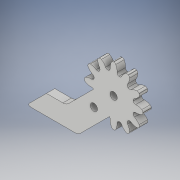
# Autodesk Inventor part: 齒輪
Saved by Autodesk Inventor 2019 (Build 230136000, 136)
## iProperties
Created: 2022-01-10
Part Number: 齒輪
Material: 一般
Document SubType Name: Modeling
Designer: 10617
Density: 1 g/cm^3
Appearance: 預設
Author: 10617
Autodesk Inventor part; units mm, degrees
ref_plane "YZ Plane" through (0, 0, 0) normal (1, 0, 0) x (0, 1, 0)
ref_plane "XZ Plane" through (0, 0, 0) normal (0, 1, 0) x (-1, 0, 0)
ref_plane "XY Plane" through (0, 0, 0) normal (0, 0, 1) x (1, 0, 0)
sketch "草圖1" plane through (0, 0, 0) normal (0, 0, 1) x (1, 0, 0)
  line L0 (35.5372, 27.5707) -> (35.6541, 27.5031)
  spline S0 degree 3 poles (35.5372, 27.5707) (35.2822, 27.7157) (34.9682, 27.7095) (34.7191, 27.5545) knots 0 0 0 0 1 1 1 1
  line L1 (35.5372, 27.5707) -> (35.2822, 27.7157) construction
  line L2 (35.2822, 27.7157) -> (34.9682, 27.7095) construction
  line L3 (34.9682, 27.7095) -> (34.7191, 27.5545) construction
  spline S1 degree 3 poles (32.2222, 25.4467) (32.622, 25.3397) (33.0418, 25.5302) (33.2243, 25.9019) knots 0.333333 0.333333 0.333333 0.333333 1 1 1 1
  line L4 (32.2222, 25.4467) -> (32.622, 25.3397) construction
  line L5 (32.622, 25.3397) -> (33.0418, 25.5302) construction
  line L6 (33.0418, 25.5302) -> (33.2243, 25.9019) construction
  spline S2 degree 3 poles (34.7191, 27.5545) (34.0759, 27.1545) (33.558, 26.5819) (33.2243, 25.9019) knots 0 0 0 0 1 1 1 1
  line L7 (34.7191, 27.5545) -> (34.0759, 27.1545) construction
  line L8 (34.0759, 27.1545) -> (33.558, 26.5819) construction
  line L9 (33.558, 26.5819) -> (33.2243, 25.9019) construction
  spline S3 degree 3 poles (31.582, 26.3419) (31.5542, 25.929) (31.8224, 25.5539) (32.2222, 25.4467) knots 0 0 0 0 0.333333 0.333333 0.333333 0.333333
  line L10 (31.582, 26.3419) -> (31.5542, 25.929) construction
  line L11 (31.5542, 25.929) -> (31.8224, 25.5539) construction
  line L12 (31.8224, 25.5539) -> (32.2222, 25.4467) construction
  spline S4 degree 3 poles (31.582, 26.3419) (31.6329, 27.0977) (31.4707, 27.8525) (31.1137, 28.5206) knots 0 0 0 0 1 1 1 1
  line L13 (31.582, 26.3419) -> (31.6329, 27.0977) construction
  line L14 (31.6329, 27.0977) -> (31.4707, 27.8525) construction
  line L15 (31.4707, 27.8525) -> (31.1137, 28.5206) construction
  spline S5 degree 3 poles (28.4693, 25.4467) (28.8691, 25.5539) (29.1373, 25.9289) (29.1096, 26.3419) knots 0.333333 0.333333 0.333333 0.333333 1 1 1 1
  line L16 (28.4693, 25.4467) -> (28.8691, 25.5539) construction
  line L17 (28.8691, 25.5539) -> (29.1373, 25.9289) construction
  line L18 (29.1373, 25.9289) -> (29.1096, 26.3419) construction
  spline S6 degree 3 poles (31.1137, 28.5206) (30.9755, 28.7793) (30.7066, 28.9417) (30.4132, 28.9436) knots 0 0 0 0 1 1 1 1
  line L19 (31.1137, 28.5206) -> (30.9755, 28.7793) construction
  line L20 (30.9755, 28.7793) -> (30.7066, 28.9417) construction
  line L21 (30.7066, 28.9417) -> (30.4132, 28.9436) construction
  spline S7 degree 3 poles (30.4132, 28.9436) (30.3683, 28.9439) (30.3233, 28.9439) (30.2782, 28.9436) knots 0 0 0 0 1 1 1 1
  line L22 (30.4132, 28.9436) -> (30.3683, 28.9439) construction
  line L23 (30.3683, 28.9439) -> (30.3233, 28.9439) construction
  line L24 (30.3233, 28.9439) -> (30.2782, 28.9436) construction
  spline S8 degree 3 poles (30.2782, 28.9436) (29.9849, 28.9418) (29.716, 28.7794) (29.5778, 28.5207) knots 0 0 0 0 1 1 1 1
  line L25 (30.2782, 28.9436) -> (29.9849, 28.9418) construction
  line L26 (29.9849, 28.9418) -> (29.716, 28.7794) construction
  line L27 (29.716, 28.7794) -> (29.5778, 28.5207) construction
  spline S9 degree 3 poles (29.5778, 28.5207) (29.2209, 27.8526) (29.0586, 27.0977) (29.1096, 26.3419) knots 0 0 0 0 1 1 1 1
  line L28 (29.5778, 28.5207) -> (29.2209, 27.8526) construction
  line L29 (29.2209, 27.8526) -> (29.0586, 27.0977) construction
  line L30 (29.0586, 27.0977) -> (29.1096, 26.3419) construction
  spline S10 degree 3 poles (27.4673, 25.9019) (27.6497, 25.5303) (28.0695, 25.3396) (28.4693, 25.4467) knots 0 0 0 0 0.333333 0.333333 0.333333 0.333333
  line L31 (27.4673, 25.9019) -> (27.6497, 25.5303) construction
  line L32 (27.6497, 25.5303) -> (28.0695, 25.3396) construction
  line L33 (28.0695, 25.3396) -> (28.4693, 25.4467) construction
  spline S11 degree 3 poles (27.4673, 25.9019) (27.1335, 26.5819) (26.6157, 27.1545) (25.9725, 27.5545) knots 0 0 0 0 1 1 1 1
  line L34 (27.4673, 25.9019) -> (27.1335, 26.5819) construction
  line L35 (27.1335, 26.5819) -> (26.6157, 27.1545) construction
  line L36 (26.6157, 27.1545) -> (25.9725, 27.5545) construction
  spline S12 degree 3 poles (24.6423, 26.7866) (24.6672, 26.0295) (24.9041, 25.2947) (25.3261, 24.6657) knots 0 0 0 0 1 1 1 1
  line L37 (24.6423, 26.7866) -> (24.6672, 26.0295) construction
  line L38 (24.6672, 26.0295) -> (24.9041, 25.2947) construction
  line L39 (24.9041, 25.2947) -> (25.3261, 24.6657) construction
  spline S13 degree 3 poles (25.9725, 27.5545) (25.7233, 27.7095) (25.4095, 27.7156) (25.1544, 27.5707) knots 0 0 0 0 1 1 1 1
  line L40 (25.9725, 27.5545) -> (25.7233, 27.7095) construction
  line L41 (25.7233, 27.7095) -> (25.4095, 27.7156) construction
  line L42 (25.4095, 27.7156) -> (25.1544, 27.5707) construction
  spline S14 degree 3 poles (25.1544, 27.5707) (25.1152, 27.5484) (25.0762, 27.5259) (25.0374, 27.5031) knots 0 0 0 0 1 1 1 1
  line L43 (25.1544, 27.5707) -> (25.1152, 27.5484) construction
  line L44 (25.1152, 27.5484) -> (25.0762, 27.5259) construction
  line L45 (25.0762, 27.5259) -> (25.0374, 27.5031) construction
  spline S15 degree 3 poles (25.0374, 27.5031) (24.7843, 27.3548) (24.6326, 27.0798) (24.6423, 26.7866) knots 0 0 0 0 1 1 1 1
  line L46 (25.0374, 27.5031) -> (24.7843, 27.3548) construction
  line L47 (24.7843, 27.3548) -> (24.6326, 27.0798) construction
  line L48 (24.6326, 27.0798) -> (24.6423, 26.7866) construction
  spline S16 degree 3 poles (36.0492, 26.7866) (36.0589, 27.0798) (35.9071, 27.3547) (35.6541, 27.5031) knots 0 0 0 0 1 1 1 1
  line L49 (36.0492, 26.7866) -> (36.0589, 27.0798) construction
  line L50 (36.0589, 27.0798) -> (35.9071, 27.3547) construction
  line L51 (35.9071, 27.3547) -> (35.6541, 27.5031) construction
  spline S17 degree 3 poles (32.2222, 11.4409) (31.8224, 11.3337) (31.5542, 10.9586) (31.582, 10.5457) knots 0.333333 0.333333 0.333333 0.333333 1 1 1 1
  line L52 (32.2222, 11.4409) -> (31.8224, 11.3337) construction
  line L53 (31.8224, 11.3337) -> (31.5542, 10.9586) construction
  line L54 (31.5542, 10.9586) -> (31.582, 10.5457) construction
  spline S18 degree 3 poles (33.2242, 10.9857) (33.0418, 11.3573) (32.622, 11.548) (32.2222, 11.4409) knots 0 0 0 0 0.333333 0.333333 0.333333 0.333333
  line L55 (33.2242, 10.9857) -> (33.0418, 11.3573) construction
  line L56 (33.0418, 11.3573) -> (32.622, 11.548) construction
  line L57 (32.622, 11.548) -> (32.2222, 11.4409) construction
  spline S19 degree 3 poles (33.2242, 10.9857) (33.558, 10.3057) (34.0759, 9.7332) (34.7191, 9.3331) knots 0 0 0 0 1 1 1 1
  line L58 (33.2242, 10.9857) -> (33.558, 10.3057) construction
  line L59 (33.558, 10.3057) -> (34.0759, 9.7332) construction
  line L60 (34.0759, 9.7332) -> (34.7191, 9.3331) construction
  spline S20 degree 3 poles (34.7191, 9.3331) (34.9682, 9.178) (35.2822, 9.172) (35.5372, 9.317) knots 0 0 0 0 1 1 1 1
  line L61 (34.7191, 9.3331) -> (34.9682, 9.178) construction
  line L62 (34.9682, 9.178) -> (35.2822, 9.172) construction
  line L63 (35.2822, 9.172) -> (35.5372, 9.317) construction
  spline S21 degree 3 poles (35.5372, 9.317) (35.5763, 9.3393) (35.6153, 9.3617) (35.6541, 9.3845) knots 0 0 0 0 1 1 1 1
  line L64 (35.5372, 9.317) -> (35.5763, 9.3393) construction
  line L65 (35.5763, 9.3393) -> (35.6153, 9.3617) construction
  line L66 (35.6153, 9.3617) -> (35.6541, 9.3845) construction
  spline S22 degree 3 poles (35.6541, 9.3845) (35.9073, 9.5329) (36.0589, 9.8078) (36.0492, 10.101) knots 0 0 0 0 1 1 1 1
  line L67 (35.6541, 9.3845) -> (35.9073, 9.5329) construction
  line L68 (35.9073, 9.5329) -> (36.0589, 9.8078) construction
  line L69 (36.0589, 9.8078) -> (36.0492, 10.101) construction
  spline S23 degree 3 poles (36.0492, 10.101) (36.0243, 10.8581) (35.7874, 11.5929) (35.3654, 12.2219) knots 0 0 0 0 1 1 1 1
  line L70 (36.0492, 10.101) -> (36.0243, 10.8581) construction
  line L71 (36.0243, 10.8581) -> (35.7874, 11.5929) construction
  line L72 (35.7874, 11.5929) -> (35.3654, 12.2219) construction
  spline S24 degree 3 poles (35.4723, 13.3172) (35.1796, 13.0246) (35.1348, 12.5657) (35.3654, 12.2219) knots 0.333333 0.333333 0.333333 0.333333 1 1 1 1
  line L73 (35.4723, 13.3172) -> (35.1796, 13.0246) construction
  line L74 (35.1796, 13.0246) -> (35.1348, 12.5657) construction
  line L75 (35.1348, 12.5657) -> (35.3654, 12.2219) construction
  spline S25 degree 3 poles (36.5676, 13.4242) (36.2239, 13.6547) (35.7651, 13.61) (35.4723, 13.3172) knots 0 0 0 0 0.333333 0.333333 0.333333 0.333333
  line L76 (36.5676, 13.4242) -> (36.2239, 13.6547) construction
  line L77 (36.2239, 13.6547) -> (35.7651, 13.61) construction
  line L78 (35.7651, 13.61) -> (35.4723, 13.3172) construction
  spline S26 degree 3 poles (36.5676, 13.4242) (37.1967, 13.0022) (37.9315, 12.7653) (38.6886, 12.7403) knots 0 0 0 0 1 1 1 1
  line L79 (36.5676, 13.4242) -> (37.1967, 13.0022) construction
  line L80 (37.1967, 13.0022) -> (37.9315, 12.7653) construction
  line L81 (37.9315, 12.7653) -> (38.6886, 12.7403) construction
  spline S27 degree 3 poles (38.6886, 12.7403) (38.9818, 12.7307) (39.2567, 12.8824) (39.405, 13.1354) knots 0 0 0 0 1 1 1 1
  line L82 (38.6886, 12.7403) -> (38.9818, 12.7307) construction
  line L83 (38.9818, 12.7307) -> (39.2567, 12.8824) construction
  line L84 (39.2567, 12.8824) -> (39.405, 13.1354) construction
  spline S28 degree 3 poles (39.405, 13.1354) (39.4279, 13.1743) (39.4504, 13.2133) (39.4726, 13.2524) knots 0 0 0 0 1 1 1 1
  line L85 (39.405, 13.1354) -> (39.4279, 13.1743) construction
  line L86 (39.4279, 13.1743) -> (39.4504, 13.2133) construction
  line L87 (39.4504, 13.2133) -> (39.4726, 13.2524) construction
  spline S29 degree 3 poles (39.4726, 13.2524) (39.6177, 13.5074) (39.6115, 13.8213) (39.4565, 14.0705) knots 0 0 0 0 1 1 1 1
  line L88 (39.4726, 13.2524) -> (39.6177, 13.5074) construction
  line L89 (39.6177, 13.5074) -> (39.6115, 13.8213) construction
  line L90 (39.6115, 13.8213) -> (39.4565, 14.0705) construction
  spline S30 degree 3 poles (39.4565, 14.0705) (39.0564, 14.7137) (38.4838, 15.2316) (37.8039, 15.5653) knots 0 0 0 0 1 1 1 1
  line L91 (39.4565, 14.0705) -> (39.0564, 14.7137) construction
  line L92 (39.0564, 14.7137) -> (38.4838, 15.2316) construction
  line L93 (38.4838, 15.2316) -> (37.8039, 15.5653) construction
  spline S31 degree 3 poles (37.3487, 16.5674) (37.2416, 16.1675) (37.4323, 15.7477) (37.8039, 15.5653) knots 0.333333 0.333333 0.333333 0.333333 1 1 1 1
  line L94 (37.3487, 16.5674) -> (37.2416, 16.1675) construction
  line L95 (37.2416, 16.1675) -> (37.4323, 15.7477) construction
  line L96 (37.4323, 15.7477) -> (37.8039, 15.5653) construction
  spline S32 degree 3 poles (35.3655, 24.6657) (35.1348, 24.3219) (35.1796, 23.863) (35.4722, 23.5704) knots 0 0 0 0 0.333333 0.333333 0.333333 0.333333
  line L97 (35.3655, 24.6657) -> (35.1348, 24.3219) construction
  line L98 (35.1348, 24.3219) -> (35.1796, 23.863) construction
  line L99 (35.1796, 23.863) -> (35.4722, 23.5704) construction
  spline S33 degree 3 poles (35.4722, 23.5704) (35.765, 23.2776) (36.2238, 23.2329) (36.5676, 23.4635) knots 0.333333 0.333333 0.333333 0.333333 1 1 1 1
  line L100 (35.4722, 23.5704) -> (35.765, 23.2776) construction
  line L101 (35.765, 23.2776) -> (36.2238, 23.2329) construction
  line L102 (36.2238, 23.2329) -> (36.5676, 23.4635) construction
  spline S34 degree 3 poles (38.6885, 24.1473) (37.9315, 24.1224) (37.1967, 23.8855) (36.5676, 23.4635) knots 0 0 0 0 1 1 1 1
  line L103 (38.6885, 24.1473) -> (37.9315, 24.1224) construction
  line L104 (37.9315, 24.1224) -> (37.1967, 23.8855) construction
  line L105 (37.1967, 23.8855) -> (36.5676, 23.4635) construction
  spline S35 degree 3 poles (39.4051, 23.7522) (39.2566, 24.0052) (38.9818, 24.157) (38.6885, 24.1473) knots 0 0 0 0 1 1 1 1
  line L106 (39.4051, 23.7522) -> (39.2566, 24.0052) construction
  line L107 (39.2566, 24.0052) -> (38.9818, 24.157) construction
  line L108 (38.9818, 24.157) -> (38.6885, 24.1473) construction
  spline S36 degree 3 poles (37.8039, 21.3223) (37.4322, 21.1399) (37.2416, 20.7201) (37.3487, 20.3203) knots 0 0 0 0 0.333333 0.333333 0.333333 0.333333
  line L109 (37.8039, 21.3223) -> (37.4322, 21.1399) construction
  line L110 (37.4322, 21.1399) -> (37.2416, 20.7201) construction
  line L111 (37.2416, 20.7201) -> (37.3487, 20.3203) construction
  spline S37 degree 3 poles (39.4726, 23.6353) (39.4504, 23.6744) (39.4278, 23.7133) (39.4051, 23.7522) knots 0 0 0 0 1 1 1 1
  line L112 (39.4726, 23.6353) -> (39.4504, 23.6744) construction
  line L113 (39.4504, 23.6744) -> (39.4278, 23.7133) construction
  line L114 (39.4278, 23.7133) -> (39.4051, 23.7522) construction
  spline S38 degree 3 poles (39.4565, 22.8171) (39.6114, 23.0663) (39.6177, 23.3802) (39.4726, 23.6353) knots 0 0 0 0 1 1 1 1
  line L115 (39.4565, 22.8171) -> (39.6114, 23.0663) construction
  line L116 (39.6114, 23.0663) -> (39.6177, 23.3802) construction
  line L117 (39.6177, 23.3802) -> (39.4726, 23.6353) construction
  spline S39 degree 3 poles (37.3487, 20.3203) (37.4558, 19.9204) (37.8309, 19.6522) (38.2439, 19.6801) knots 0.333333 0.333333 0.333333 0.333333 1 1 1 1
  line L118 (37.3487, 20.3203) -> (37.4558, 19.9204) construction
  line L119 (37.4558, 19.9204) -> (37.8309, 19.6522) construction
  line L120 (37.8309, 19.6522) -> (38.2439, 19.6801) construction
  spline S40 degree 3 poles (37.8039, 21.3223) (38.4838, 21.6561) (39.0564, 22.174) (39.4565, 22.8171) knots 0 0 0 0 1 1 1 1
  line L121 (37.8039, 21.3223) -> (38.4838, 21.6561) construction
  line L122 (38.4838, 21.6561) -> (39.0564, 22.174) construction
  line L123 (39.0564, 22.174) -> (39.4565, 22.8171) construction
  spline S41 degree 3 poles (40.4226, 19.2117) (39.7545, 19.5687) (38.9996, 19.731) (38.2439, 19.6801) knots 0 0 0 0 1 1 1 1
  line L124 (40.4226, 19.2117) -> (39.7545, 19.5687) construction
  line L125 (39.7545, 19.5687) -> (38.9996, 19.731) construction
  line L126 (38.9996, 19.731) -> (38.2439, 19.6801) construction
  spline S42 degree 3 poles (40.8455, 18.3762) (40.8458, 18.4213) (40.8458, 18.4663) (40.8455, 18.5113) knots 0 0 0 0 1 1 1 1
  line L127 (40.8455, 18.3762) -> (40.8458, 18.4213) construction
  line L128 (40.8458, 18.4213) -> (40.8458, 18.4663) construction
  line L129 (40.8458, 18.4663) -> (40.8455, 18.5113) construction
  spline S43 degree 3 poles (40.8455, 18.5113) (40.8436, 18.8047) (40.6813, 19.0735) (40.4226, 19.2117) knots 0 0 0 0 1 1 1 1
  line L130 (40.8455, 18.5113) -> (40.8436, 18.8047) construction
  line L131 (40.8436, 18.8047) -> (40.6813, 19.0735) construction
  line L132 (40.6813, 19.0735) -> (40.4226, 19.2117) construction
  spline S44 degree 3 poles (40.4226, 17.6758) (40.6814, 17.8141) (40.8437, 18.0829) (40.8455, 18.3762) knots 0 0 0 0 1 1 1 1
  line L133 (40.4226, 17.6758) -> (40.6814, 17.8141) construction
  line L134 (40.6814, 17.8141) -> (40.8437, 18.0829) construction
  line L135 (40.8437, 18.0829) -> (40.8455, 18.3762) construction
  spline S45 degree 3 poles (38.2439, 17.2076) (38.9996, 17.1567) (39.7545, 17.3189) (40.4226, 17.6758) knots 0 0 0 0 1 1 1 1
  line L136 (38.2439, 17.2076) -> (38.9996, 17.1567) construction
  line L137 (38.9996, 17.1567) -> (39.7545, 17.3189) construction
  line L138 (39.7545, 17.3189) -> (40.4226, 17.6758) construction
  spline S46 degree 3 poles (38.2439, 17.2076) (37.8309, 17.2353) (37.4559, 16.9672) (37.3487, 16.5674) knots 0 0 0 0 0.333333 0.333333 0.333333 0.333333
  line L139 (38.2439, 17.2076) -> (37.8309, 17.2353) construction
  line L140 (37.8309, 17.2353) -> (37.4559, 16.9672) construction
  line L141 (37.4559, 16.9672) -> (37.3487, 16.5674) construction
  spline S47 degree 3 poles (35.3655, 24.6657) (35.7875, 25.2947) (36.0243, 26.0295) (36.0492, 26.7866) knots 0 0 0 0 1 1 1 1
  line L142 (35.3655, 24.6657) -> (35.7875, 25.2947) construction
  line L143 (35.7875, 25.2947) -> (36.0243, 26.0295) construction
  line L144 (36.0243, 26.0295) -> (36.0492, 26.7866) construction
  arc A0 (12.1679, 7.1654) -> (14.2893, 8.0441) centre (12.1679, 10.1655) ccw
  arc A1 (0.0524, 0.9447) -> (0.4048, 0.0944) centre (0.4031, 0.5919) ccw
  arc A2 (16.4106, 0.0943) -> (18.5319, 0.9731) centre (16.4105, 3.0945) ccw
  line L145 (14.2893, 8.0441) -> (23.1584, 16.9132)
  line L146 (6.2687, 7.1655) -> (12.1679, 7.1654)
  line L147 (6.2687, 7.1655) -> (0.0524, 0.9447)
  line L148 (0.4048, 0.0944) -> (16.4106, 0.0943)
  line L149 (18.5319, 0.9731) -> (28.8152, 11.2564)
  spline S48 degree 3 poles (30.2783, 7.944) (30.3232, 7.9437) (30.3683, 7.9438) (30.4133, 7.944) knots 0 0 0 0 1 1 1 1
  line L150 (30.2783, 7.944) -> (30.3232, 7.9437) construction
  line L151 (30.3232, 7.9437) -> (30.3683, 7.9438) construction
  line L152 (30.3683, 7.9438) -> (30.4133, 7.944) construction
  spline S49 degree 3 poles (30.4133, 7.944) (30.7067, 7.9459) (30.9755, 8.1082) (31.1138, 8.367) knots 0 0 0 0 1 1 1 1
  line L153 (30.4133, 7.944) -> (30.7067, 7.9459) construction
  line L154 (30.7067, 7.9459) -> (30.9755, 8.1082) construction
  line L155 (30.9755, 8.1082) -> (31.1138, 8.367) construction
  spline S50 degree 3 poles (31.1138, 8.367) (31.4707, 9.0351) (31.6329, 9.79) (31.582, 10.5457) knots 0 0 0 0 1 1 1 1
  line L156 (31.1138, 8.367) -> (31.4707, 9.0351) construction
  line L157 (31.4707, 9.0351) -> (31.6329, 9.79) construction
  line L158 (31.6329, 9.79) -> (31.582, 10.5457) construction
  circle A3 centre (23.2746, 11.3728) radius 1.3
  spline S51 degree 3 poles (29.1096, 10.5457) (29.1277, 10.8155) (29.0188, 11.0784) (28.8152, 11.2564) knots 0 0 0 0 1 1 1 1
  line L159 (29.1096, 10.5457) -> (29.1277, 10.8155) construction
  line L160 (29.1277, 10.8155) -> (29.0188, 11.0784) construction
  line L161 (29.0188, 11.0784) -> (28.8152, 11.2564) construction
  spline S52 degree 3 poles (29.5778, 8.367) (29.716, 8.1083) (29.9849, 7.9459) (30.2783, 7.944) knots 0 0 0 0 1 1 1 1
  line L162 (29.5778, 8.367) -> (29.716, 8.1083) construction
  line L163 (29.716, 8.1083) -> (29.9849, 7.9459) construction
  line L164 (29.9849, 7.9459) -> (30.2783, 7.944) construction
  spline S53 degree 3 poles (29.1096, 10.5457) (29.0586, 9.7899) (29.2209, 9.0351) (29.5778, 8.367) knots 0 0 0 0 1 1 1 1
  line L165 (29.1096, 10.5457) -> (29.0586, 9.7899) construction
  line L166 (29.0586, 9.7899) -> (29.2209, 9.0351) construction
  line L167 (29.2209, 9.0351) -> (29.5778, 8.367) construction
  spline S54 degree 3 poles (25.2193, 23.5703) (25.512, 23.863) (25.5567, 24.3219) (25.3261, 24.6657) knots 0.333333 0.333333 0.333333 0.333333 1 1 1 1
  line L168 (25.2193, 23.5703) -> (25.512, 23.863) construction
  line L169 (25.512, 23.863) -> (25.5567, 24.3219) construction
  line L170 (25.5567, 24.3219) -> (25.3261, 24.6657) construction
  circle A4 centre (30.3458, 18.4439) radius 1.3
  spline S55 degree 3 poles (24.1239, 23.4634) (24.4676, 23.2329) (24.9266, 23.2776) (25.2193, 23.5703) knots 0 0 0 0 0.333333 0.333333 0.333333 0.333333
  line L171 (24.1239, 23.4634) -> (24.4676, 23.2329) construction
  line L172 (24.4676, 23.2329) -> (24.9266, 23.2776) construction
  line L173 (24.9266, 23.2776) -> (25.2193, 23.5703) construction
  spline S56 degree 3 poles (24.1239, 23.4634) (23.4948, 23.8854) (22.7601, 24.1224) (22.003, 24.1472) knots 0 0 0 0 1 1 1 1
  line L174 (24.1239, 23.4634) -> (23.4948, 23.8854) construction
  line L175 (23.4948, 23.8854) -> (22.7601, 24.1224) construction
  line L176 (22.7601, 24.1224) -> (22.003, 24.1472) construction
  spline S57 degree 3 poles (22.003, 24.1472) (21.7098, 24.1569) (21.4348, 24.0053) (21.2865, 23.7522) knots 0 0 0 0 1 1 1 1
  line L177 (22.003, 24.1472) -> (21.7098, 24.1569) construction
  line L178 (21.7098, 24.1569) -> (21.4348, 24.0053) construction
  line L179 (21.4348, 24.0053) -> (21.2865, 23.7522) construction
  spline S58 degree 3 poles (21.2865, 23.7522) (21.2636, 23.7133) (21.2412, 23.6744) (21.2189, 23.6353) knots 0 0 0 0 1 1 1 1
  line L180 (21.2865, 23.7522) -> (21.2636, 23.7133) construction
  line L181 (21.2636, 23.7133) -> (21.2412, 23.6744) construction
  line L182 (21.2412, 23.6744) -> (21.2189, 23.6353) construction
  spline S59 degree 3 poles (23.3428, 20.3202) (23.4499, 20.7201) (23.2592, 21.1399) (22.8876, 21.3223) knots 0.333333 0.333333 0.333333 0.333333 1 1 1 1
  line L183 (23.3428, 20.3202) -> (23.4499, 20.7201) construction
  line L184 (23.4499, 20.7201) -> (23.2592, 21.1399) construction
  line L185 (23.2592, 21.1399) -> (22.8876, 21.3223) construction
  spline S60 degree 3 poles (22.4476, 19.68) (22.8606, 19.6522) (23.2356, 19.9204) (23.3428, 20.3202) knots 0 0 0 0 0.333333 0.333333 0.333333 0.333333
  line L186 (22.4476, 19.68) -> (22.8606, 19.6522) construction
  line L187 (22.8606, 19.6522) -> (23.2356, 19.9204) construction
  line L188 (23.2356, 19.9204) -> (23.3428, 20.3202) construction
  spline S61 degree 3 poles (21.2351, 22.8171) (21.6352, 22.174) (22.2077, 21.656) (22.8876, 21.3223) knots 0 0 0 0 1 1 1 1
  line L189 (21.2351, 22.8171) -> (21.6352, 22.174) construction
  line L190 (21.6352, 22.174) -> (22.2077, 21.656) construction
  line L191 (22.2077, 21.656) -> (22.8876, 21.3223) construction
  spline S62 degree 3 poles (23.1584, 16.9132) (22.9804, 17.1169) (22.7174, 17.2258) (22.4477, 17.2076) knots 0 0 0 0 1 1 1 1
  line L192 (23.1584, 16.9132) -> (22.9804, 17.1169) construction
  line L193 (22.9804, 17.1169) -> (22.7174, 17.2258) construction
  line L194 (22.7174, 17.2258) -> (22.4477, 17.2076) construction
  spline S63 degree 3 poles (22.4476, 19.68) (21.6919, 19.731) (20.937, 19.5688) (20.2689, 19.2118) knots 0 0 0 0 1 1 1 1
  line L195 (22.4476, 19.68) -> (21.6919, 19.731) construction
  line L196 (21.6919, 19.731) -> (20.937, 19.5688) construction
  line L197 (20.937, 19.5688) -> (20.2689, 19.2118) construction
  spline S64 degree 3 poles (19.846, 18.5114) (19.8457, 18.4663) (19.8457, 18.4213) (19.846, 18.3763) knots 0 0 0 0 1 1 1 1
  line L198 (19.846, 18.5114) -> (19.8457, 18.4663) construction
  line L199 (19.8457, 18.4663) -> (19.8457, 18.4213) construction
  line L200 (19.8457, 18.4213) -> (19.846, 18.3763) construction
  spline S65 degree 3 poles (20.2689, 19.2118) (20.0101, 19.0735) (19.8479, 18.8047) (19.846, 18.5114) knots 0 0 0 0 1 1 1 1
  line L201 (20.2689, 19.2118) -> (20.0101, 19.0735) construction
  line L202 (20.0101, 19.0735) -> (19.8479, 18.8047) construction
  line L203 (19.8479, 18.8047) -> (19.846, 18.5114) construction
  spline S66 degree 3 poles (20.2689, 17.6758) (20.937, 17.3189) (21.6919, 17.1566) (22.4477, 17.2076) knots 0 0 0 0 1 1 1 1
  line L204 (20.2689, 17.6758) -> (20.937, 17.3189) construction
  line L205 (20.937, 17.3189) -> (21.6919, 17.1566) construction
  line L206 (21.6919, 17.1566) -> (22.4477, 17.2076) construction
  spline S67 degree 3 poles (19.846, 18.3763) (19.8479, 18.0829) (20.0102, 17.8141) (20.2689, 17.6758) knots 0 0 0 0 1 1 1 1
  line L207 (19.846, 18.3763) -> (19.8479, 18.0829) construction
  line L208 (19.8479, 18.0829) -> (20.0102, 17.8141) construction
  line L209 (20.0102, 17.8141) -> (20.2689, 17.6758) construction
  spline S68 degree 3 poles (21.2189, 23.6353) (21.074, 23.3801) (21.08, 23.0663) (21.2351, 22.8171) knots 0 0 0 0 1 1 1 1
  line L210 (21.2189, 23.6353) -> (21.074, 23.3801) construction
  line L211 (21.074, 23.3801) -> (21.08, 23.0663) construction
  line L212 (21.08, 23.0663) -> (21.2351, 22.8171) construction
  point P0 (0, 0)
  constraints: 12 end point, 6 point on circle, 5 centre point, 207 other
extrude "擠出1" add sketch "草圖1" along normal blind 3
